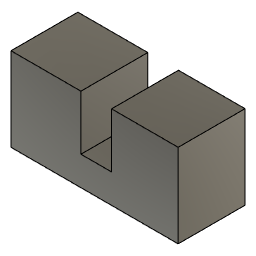
eye_blinker_slider_stopper (Autodesk Fusion 360 design; units mm, degrees)
Autodesk Fusion 360 part; units mm, degrees
sketch "Sketch1" plane through (0, 0, 0) normal (0, 1, 0) x (1, 0, 0)
  line L0 (0, 0) -> (6, 0)
  line L1 (6, 0) -> (6, -3)
  line L2 (6, -3) -> (0, -3)
  line L3 (0, -3) -> (0, 0)
  dimension "d1" = 6
  dimension "d2" = 3
  constraint horizontal L0
  constraint vertical L1
  constraint horizontal L2
  constraint vertical L3
  constraint coincident L0.start L3.end
  measures "d1" distance of L0.start L0.end
  measures "d2" distance of L0.start L2.end
extrude "Extrude1" add sketch "Sketch1" along normal blind 2.4
sketch "Sketch2" plane through (0, 0, 0) normal (0, -1, 0) x (1, 0, 0)
  line L0 (6, 3) -> (0, 3)
  line L1 (0, 3) -> (0, 0)
  line L2 (0, 0) -> (6, 0)
  line L3 (6, 0) -> (6, 3)
  line L4 (6, 3) -> (6, 1.04)
  line L5 (6, 3) -> (3.61, 3)
  line L6 (0, 3) -> (2.51, 3)
  line L7 (0, 3) -> (0, 1.04)
  line L8 (2.51, 3) -> (3.61, 3)
  line L9 (3.61, 3) -> (3.61, 1.04)
  line L10 (3.61, 1.04) -> (2.51, 1.04)
  line L11 (2.51, 1.04) -> (2.51, 3)
  dimension "d5" = 1.96
  dimension "d6" = 2.39
  dimension "d7" = 2.51
  dimension "d8" = 1.96
  dimension "d9" = 1.96
  constraint coincident L0.start L3.end
  constraint perpendicular L0 L4
  constraint perpendicular L4 L5
  constraint coincident L0.end L1.start
  constraint perpendicular L1 L6
  constraint perpendicular L0 L7
  constraint horizontal L8
  constraint vertical L9
  constraint horizontal L10
  constraint vertical L11
  measures "d5" distance of L0.start L4.end
  measures "d6" distance of L0.start L5.end
  measures "d7" distance of L0.end L6.end
  measures "d8" distance of L0.end L7.end
  measures "d9" distance of L6.end L10.end
extrude "Extrude2" cut sketch "Sketch2" against normal blind 4.6 contours L0 L8 L9 L10 L11
